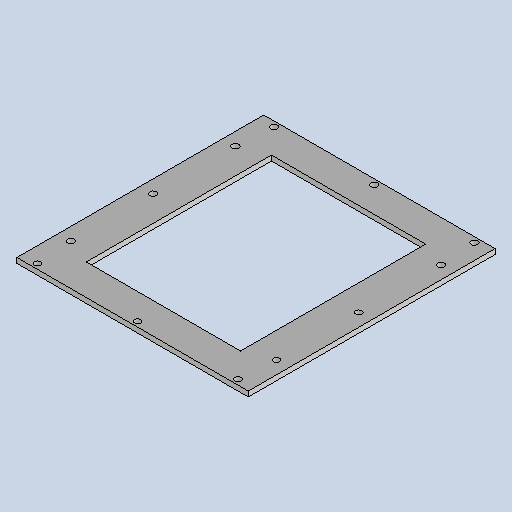
# Autodesk Inventor part: NVPH-305 main flange
Saved by Autodesk Inventor 2025 (Build 290162010, 162A)
## iProperties
Created: 2024-12-03
Part Number: NVPH-305 main flange
Material: Generic
Document SubType Name: Sheet Metal
Designer: user
Density: 1 g/cm^3
Flat Pattern Width: 45 cm
Flat Pattern Length: 48 cm
Flat Pattern Area: 2160 cm^2
Sheet Metal Rule: Default
Sheet Metal Width: 450,000 mm
Sheet Metal Length: 480,000 mm
Sheet Metal Area: 216000,000 mm^2
Appearance: Default
Mass: 1065.05 g
Surface Area: 2495.55 cm^2
Volume: 1065.05 cm^3
Author: user
Autodesk Inventor part; units mm, degrees
ref_plane "YZ Plane" through (0, 0, 0) normal (1, 0, 0) x (0, 1, 0)
ref_plane "XZ Plane" through (0, 0, 0) normal (0, 1, 0) x (-1, 0, 0)
ref_plane "XY Plane" through (0, 0, 0) normal (0, 0, 1) x (1, 0, 0)
sketch "Sketch3" plane through (0, 0, 0) normal (0, 0, 1) x (1, 0, 0)
  line L0 (225, 240) -> (-225, 240)
  line L1 (-225, 240) -> (-225, -240)
  line L2 (-225, -240) -> (225, -240)
  line L3 (225, -240) -> (225, 240)
  line L4 (225, 240) -> (-225, -240) construction
  line L5 (-225, 240) -> (225, -240) construction
  line L6 (150, 180) -> (-150, 180)
  line L7 (-150, 180) -> (-150, -180)
  line L8 (-150, -180) -> (150, -180)
  line L9 (150, -180) -> (150, 180)
  line L10 (150, 180) -> (-150, -180) construction
  line L11 (-150, 180) -> (150, -180) construction
  point P0 (0, 0)
  dimension "d22" = 450
  dimension "d23" = 480
  dimension "d24" = 300
  dimension "d25" = 360
  measures "d22" distance of L2.end L1.end
  measures "d23" distance of L1.end L0.end
  measures "d24" distance of L8.end L7.end
  measures "d25" distance of L7.end L6.end
extrude "Plate3" add sketch "Sketch3" along normal blind 10
sketch "Sketch4" plane through (0, 0, 0) normal (0, 0, -1) x (-1, 0, 0)
  circle A0 centre (0, 230) radius 6.5 projected
  circle A1 centre (195, 230) radius 6.5 projected
  circle A2 centre (-195, 230) radius 6.5 projected
  circle A3 centre (-200, 160) radius 6.5 projected
  circle A4 centre (-200, 0) radius 6 projected
  circle A5 centre (-200, -160) radius 6 projected
  circle A6 centre (-195, -230) radius 6 projected
  circle A7 centre (0, -230) radius 6 projected
  circle A8 centre (195, -230) radius 6 projected
  circle A9 centre (200, -160) radius 6.5 projected
  circle A10 centre (200, 0) radius 6.5 projected
  circle A11 centre (200, 160) radius 6.5 projected
  point P0 (0, 0)
extrude "Cut1" cut sketch "Sketch4" against normal blind 10
equation "\"d26\" = Thickness"
equation "\"d18\" = Thickness"
equation "\"BendReliefDepth\" = 0.5 * Thickness"
equation "\"Thickness\" = 10"
body "Solid2"
